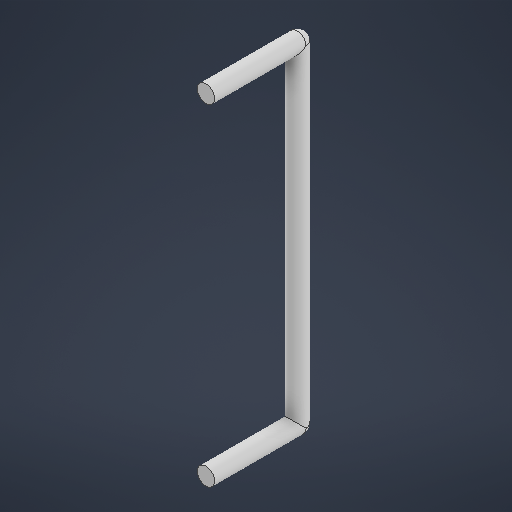
# Autodesk Inventor part: Union_Poleas
Saved by Autodesk Inventor 2026.2 (Build 302298010, 298A)
## iProperties
Created: 2026-04-28
Part Number: Union_Poleas
Material: Genérico
Document SubType Name: Modeling
Designer: agusb
Density: 1 g/cm^3
Appearance: Valor por defecto
Author: agusb
Autodesk Inventor part; units mm, degrees
ref_plane "YZ Plane" through (0, 0, 0) normal (1, 0, 0) x (0, 1, 0)
ref_plane "XZ Plane" through (0, 0, 0) normal (0, 1, 0) x (-1, 0, 0)
ref_plane "XY Plane" through (0, 0, 0) normal (0, 0, 1) x (1, 0, 0)
sketch "Boceto1" plane through (0, 0, 0) normal (0, 1, 0) x (-1, 0, 0)
  line L0 (0, 0) -> (-100, 0)
  line L1 (-100, 0) -> (-100, -100)
  line L2 (-100, -100) -> (0, -100)
  line L3 (0, -100) -> (0, 0)
  dimension "d0" = 100
  dimension "d1" = 100
  constraints: 8 end point, 2 parallel, 1 horizontal, 1 perpendicular
  measures "d0" distance of L2.end L1.end
  measures "d1" distance of L1.end L0.end
extrude "Extrusión1" add sketch "Boceto1" along normal blind 2020
sketch "Boceto2" plane through (0, 0, 0) normal (0, 0, 1) x (1, 0, 0)
  line L0 (100, 2020) -> (0, 2020) projected
  line L1 (100, 0) -> (100, 2020) projected
  line L2 (0, 2020) -> (100, 2020)
  line L3 (100, 2020) -> (100, 1920)
  line L4 (100, 1920) -> (0, 1920)
  line L5 (0, 1920) -> (0, 2020)
  line L6 (0, 0) -> (100, 0)
  line L7 (100, 0) -> (100, 100)
  line L8 (100, 100) -> (0, 100)
  line L9 (0, 100) -> (0, 0)
  dimension "d4" = 100
  dimension "d5" = 100
  constraints: 16 end point, 4 parallel, 2 horizontal, 2 perpendicular, 2 point on line
  measures "d4" distance of L2.end L3.end
  measures "d5" distance of L7.end L6.end
extrude "Extrusión2" add sketch "Boceto2" along normal blind 480
fillet "Empalme1" radius 50 1 edges at (0, 2020, 190)
fillet "Empalme2" radius 50 1 edges at (100, 2020, 190)
fillet "Empalme3" radius 50 1 edges at (0, 1920, 240)
fillet "Empalme4" radius 50 1 edges at (100, 1920, 240)
fillet "Empalme5" radius 50 3 edges at (14.6447, 2005.3553, -100) (100, 985.0003, -100) (0, 985, -100)
fillet "Empalme6" radius 50 1 edges at (85.3555, 0, -85.3555)
fillet "Empalme7" radius 50 1 edges at (0, 100, 240)
fillet "Empalme8" radius 50 1 edges at (100, 100, 240)
fillet "Empalme9" radius 50 2 edges at (0, 75, 0) (0, 1944.9997, 0)
fillet "Empalme10" radius 50 1 edges at (100, 75.0003, 0)
